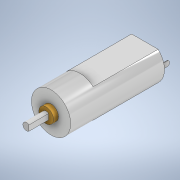
# Autodesk Inventor part: DriveMotorV1
Saved by Autodesk Inventor 2020 (Build 240168000, 168)
## iProperties
Created: 2023-11-25
Part Number: DriveMotorV1
Material: Motor
Document SubType Name: Modeling
Designer: smz3rm
Density: 3.93364 g/cm^3
Appearance: Default
Mass: 27.6 g
Surface Area: 24.374 cm^2
Volume: 7.01639 cm^3
Author: smz3rm
Autodesk Inventor part; units mm, degrees
ref_plane "YZ Plane" through (0, 0, 0) normal (1, 0, 0) x (0, 1, 0)
ref_plane "XZ Plane" through (0, 0, 0) normal (0, 1, 0) x (-1, 0, 0)
ref_plane "XY Plane" through (0, 0, 0) normal (0, 0, 1) x (1, 0, 0)
sketch "Sketch3" plane through (0, 0, 0) normal (0, 0, 1) x (1, 0, 0)
  circle A0 centre (0, 0) radius 8
  dimension "d1" = 16
  constraints: 1 centre point, 1 coincident
  measures "d1" diameter of A0
extrude "Extrusion1" add sketch "Sketch3" against normal blind 11.75
sketch "Sketch4" plane through (0, 0, -11.75) normal (0, 0, -1) x (-1, 0, 0)
  line L0 (-5.4028, 5.9) -> (5.4028, 5.9)
  circle A0 centre (0, 0) radius 8 projected
  line L1 (-5.4028, -5.9) -> (5.4028, -5.9)
  line L2 (0, 5.9) -> (0, -5.9)
  dimension "d6" = 11.8
  constraints: 6 end point, 4 point on circle, 3 midpoint, 1 coincident, 1 horizontal, 1 parallel
  measures "d6" distance between parallel lines of L1 L0
extrude "Extrusion2" add sketch "Sketch4" along normal blind 26.5 contours L0 L2 L1 A0 | L0 A0 L1 L2
sketch "Sketch5" plane through (0, 0, 0) normal (0, 0, 1) x (1, 0, 0)
  circle A0 centre (0, 0) radius 3
  dimension "d9" = 6
  constraints: 1 centre point, 1 coincident
  measures "d9" diameter of A0
extrude "Extrusion3" add sketch "Sketch5" along normal blind 2
sketch "Sketch6" plane through (0, 0, 2) normal (0, 0, 1) x (1, 0, 0)
  circle A0 centre (0, 0) radius 1.5
  line L0 (0, -11.2) -> (0, 11.2) projected
  line L1 (1, 1.118) -> (1, -1.118)
  dimension "d12" = 3
  dimension "d13" = 1
  constraints: 2 end point, 2 point on circle, 1 centre point, 1 coincident, 1 vertical
  measures "d12" diameter of A0
  measures "d13" distance between parallel lines of L0 L1
extrude "Extrusion4" add sketch "Sketch6" along normal blind 8 contours L1 A0 L0 | L0 A0
sketch "Sketch7" plane through (0, 0, -38.25) normal (0, 0, -1) x (-1, 0, 0)
  circle A0 centre (0, 0) radius 2.95
  dimension "d16" = 5.9
  constraints: 1 centre point, 1 coincident
  measures "d16" diameter of A0
extrude "Extrusion5" add sketch "Sketch7" along normal blind 1.5
sketch "Sketch10" plane through (0, 0, -38.25) normal (0, 0, -1) x (-1, 0, 0)
  line L0 (-6.5, -1) -> (-6.25, -1)
  line L1 (-6.25, -1) -> (-6.25, 1)
  line L2 (-6.25, 1) -> (-6.5, 1)
  line L3 (-6.5, 1) -> (-6.5, -1)
  line L4 (-6.5, -1) -> (-6.25, 1) construction
  line L5 (-6.25, -1) -> (-6.5, 1) construction
  line L6 (11.2, 0) -> (-11.2, 0) projected
  line L7 (0, -11.2) -> (0, 11.2) projected
  line L8 (6.5, -1) -> (6.25, -1)
  line L9 (6.25, -1) -> (6.25, 1)
  line L10 (6.25, 1) -> (6.5, 1)
  line L11 (6.5, 1) -> (6.5, -1)
  point P0 (0, 0)
  point P1 (-6.375, 0)
  point P2 (-6.375, 0)
  dimension "d23" = 0.25
  dimension "d24" = 2
  dimension "d25" = 13
  constraints: 20 end point, 4 symmetric about line, 3 midpoint, 2 parallel, 1 horizontal, 1 perpendicular, 1 point on line
  measures "d23" distance of L2.end L1.end
  measures "d24" distance of L0.end L1.end
  measures "d25" distance between parallel lines of L11 L3
extrude "Extrusion7" add sketch "Sketch10" along normal blind 3.5
fillet "Fillet2" radius 0.8 4 edges at (-6.375, 1, -41.75) (-6.375, -1, -41.75) (6.375, 1, -41.75) (6.375, -1, -41.75)
body "Solid1"
